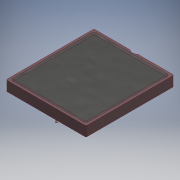
# Autodesk Inventor part: Semiconductor_RadiationDiode
Saved by Autodesk Inventor 2018 (Build 220112000, 112)
## iProperties
Created: 2018-01-16
Part Number: Semiconductor_RadiationDiode
Material: ABS Plastic
Document SubType Name: Modeling
Designer: Bradley
Mass: 0.33228 g
Surface Area: 5.66161 cm^2
Volume: 0.313472 cm^3
Density: 1.06 g/cm^3
Appearance: Smooth - Dark Maroon
Stock Number: X100-7 SMD
Author: Bradley
Autodesk Inventor part; units mm, degrees
ref_plane "YZ Plane" through (0, 0, 0) normal (1, 0, 0) x (0, 1, 0)
ref_plane "XZ Plane" through (0, 0, 0) normal (0, 1, 0) x (-1, 0, 0)
ref_plane "XY Plane" through (0, 0, 0) normal (0, 0, 1) x (1, 0, 0)
sketch "Sketch1" plane through (0, 0, 0) normal (0, 0, 1) x (1, 0, 0)
  line L0 (-7.5, -8.25) -> (7.5, -8.25)
  line L1 (7.5, -8.25) -> (7.5, 8.25)
  line L2 (7.5, 8.25) -> (-7.5, 8.25)
  line L3 (-7.5, 8.25) -> (-7.5, -8.25)
  line L4 (-7.5, -8.25) -> (7.5, 8.25) construction
  line L5 (7.5, -8.25) -> (-7.5, 8.25) construction
  arc A0 (-0.7141, 8.25) -> (0.7141, 8.25) centre (0, 8.95) ccw
  line L6 (0, 7.95) -> (0, 8.25) construction
  point P0 (0, 0)
  dimension "d0" = 15
  dimension "d1" = 16.5
  dimension "d23" = 0.3
  dimension "d24" = 1
  constraints: 14 end point, 3 midpoint, 3 point on circle, 2 parallel, 2 perpendicular, 2 point on line, 1 centre point, 1 horizontal
  measures "d0" distance of L2.end L1.end
  measures "d1" distance of L1.end L0.end
  measures "d23" distance of L6.start L6.end
  measures "d24" radius of A0
extrude "Extrusion1" add sketch "Sketch1" along normal mid plane 2.1 contours L3 L2 A0 L1 L0
fillet "Fillet1" radius 0.2 6 edges at (-7.5, 8.25, 0) (7.5, 8.25, 0) (7.5, -8.25, 0) (-7.5, -8.25, 0) (-0.7141, 8.25, 0) (0.7141, 8.25, 0)
sketch "Sketch2" plane through (0, 0, 1.05) normal (0, 0, 1) x (1, 0, 0)
  arc A0 (-7.5, -8.05) -> (-7.3, -8.25) centre (-7.3, -8.05) ccw projected
  line L0 (-7.3, -8.25) -> (7.3, -8.25) projected
  arc A1 (7.3, -8.25) -> (7.5, -8.05) centre (7.3, -8.05) ccw projected
  line L1 (7.5, -8.05) -> (7.5, 8.05) projected
  arc A2 (7.5, 8.05) -> (7.3, 8.25) centre (7.3, 8.05) ccw projected
  line L2 (7.3, 8.25) -> (0.7937, 8.25) projected
  arc A3 (-7.3, 8.25) -> (-7.5, 8.05) centre (-7.3, 8.05) ccw projected
  line L3 (-7.5, 8.05) -> (-7.5, -8.05) projected
  line L4 (6.6, -7.85) -> (-6.6, -7.85)
  line L5 (-7.1, -7.35) -> (-7.1, 7.35)
  line L6 (-6.6, 7.85) -> (6.6, 7.85)
  line L7 (7.1, 7.35) -> (7.1, -7.35)
  line L8 (7.1, -7.85) -> (-7.1, 7.85) construction
  line L9 (-7.1, -7.85) -> (7.1, 7.85) construction
  arc A4 (-6.6, 7.85) -> (-7.1, 7.35) centre (-6.6, 7.35) ccw
  arc A5 (7.1, 7.35) -> (6.6, 7.85) centre (6.6, 7.35) ccw
  arc A6 (6.6, -7.85) -> (7.1, -7.35) centre (6.6, -7.35) ccw
  arc A7 (-7.1, -7.35) -> (-6.6, -7.85) centre (-6.6, -7.35) ccw
  arc A8 (-0.6614, 8.2) -> (0.6614, 8.2) centre (0, 8.95) ccw projected
  line L10 (-0.7937, 8.25) -> (-7.3, 8.25) projected
  arc A9 (0.7937, 8.25) -> (0.6614, 8.2) centre (0.7937, 8.05) ccw projected
  arc A10 (-0.6614, 8.2) -> (-0.7937, 8.25) centre (-0.7937, 8.05) ccw projected
  point P0 (0, 0)
  dimension "d5" = 0.4
  dimension "d6" = 0.4
  dimension "d7" = 0.5
  constraints: 12 end point, 8 point on circle, 8 point on line, 8 tangent, 4 centre point, 3 equal radius, 2 midpoint, 2 parallel, 1 horizontal, 1 perpendicular
  measures "d5" distance between parallel lines of L6 L2
  measures "d6" distance between parallel lines of L3 L5
  measures "d7" radius of A4
extrude "Extrusion2" cut sketch "Sketch2" against normal blind 0.1 contours L4 A7 L5 A4 L6 A5 L7 A6
fillet "Fillet2" radius 1 8 edges at (-7.1, 0, 0.95) (-6.9536, 7.7036, 0.95) (0, 7.85, 0.95) (6.9536, 7.7036, 0.95) (7.1, 0, 0.95) (6.9536, -7.7036, 0.95) (0, -7.85, 0.95) (-6.9536, -7.7036, 0.95)
sketch "Sketch4" plane through (0, 0, -1.05) normal (0, 0, -1) x (-1, 0, 0)
  arc A0 (-0.6614, 8.2) -> (-0.7937, 8.25) centre (-0.7937, 8.05) ccw projected
  line L0 (-0.7937, 8.25) -> (-7.3, 8.25) projected
  arc A1 (-7.3, 8.25) -> (-7.5, 8.05) centre (-7.3, 8.05) ccw projected
  line L1 (-7.5, 8.05) -> (-7.5, -8.05) projected
  arc A2 (-7.5, -8.05) -> (-7.3, -8.25) centre (-7.3, -8.05) ccw projected
  line L2 (-7.3, -8.25) -> (7.3, -8.25) projected
  arc A3 (7.3, -8.25) -> (7.5, -8.05) centre (7.3, -8.05) ccw projected
  line L3 (7.5, -8.05) -> (7.5, 8.05) projected
  arc A4 (7.5, 8.05) -> (7.3, 8.25) centre (7.3, 8.05) ccw projected
  line L4 (7.3, 8.25) -> (0.7937, 8.25) projected
  arc A5 (0.7937, 8.25) -> (0.6614, 8.2) centre (0.7937, 8.05) ccw projected
  arc A6 (-0.6614, 8.2) -> (0.6614, 8.2) centre (0, 8.95) ccw projected
  line L5 (-6.8, -7.55) -> (6.8, -7.55)
  line L6 (6.8, -7.55) -> (6.8, 7.55)
  line L7 (6.8, 7.55) -> (-6.8, 7.55)
  line L8 (-6.8, 7.55) -> (-6.8, -7.55)
  line L9 (-6.8, -7.55) -> (6.8, 7.55) construction
  line L10 (6.8, -7.55) -> (-6.8, 7.55) construction
  point P0 (0, 0)
  dimension "d25" = 13.6
  dimension "d26" = 15.1
  constraints: 12 end point, 2 midpoint, 2 parallel, 1 horizontal, 1 perpendicular
  measures "d25" distance of L7.end L6.end
  measures "d26" distance of L6.end L5.end
extrude "Extrusion4" cut sketch "Sketch4" against normal blind 0.25
sketch "Sketch5" plane through (0, 0, -1.05) normal (0, 0, -1) x (-1, 0, 0)
  circle A0 centre (0, 6.25) radius 0.225
  circle A1 centre (0, -6.25) radius 0.225
  line L0 (0, 6.25) -> (0, -6.25) construction
  point P0 (0, 0)
  point P1 (0, 0)
  dimension "d29" = 0.45
  dimension "d30" = 12.5
  constraints: 2 centre point, 2 end point, 1 coincident, 1 equal radius, 1 midpoint, 1 vertical
  measures "d29" diameter of A0
  measures "d30" distance of L0.start L0.end
extrude "Extrusion5" add sketch "Sketch5" along normal blind 2
equation "\"d6\" = d5"
body "Solid1"
